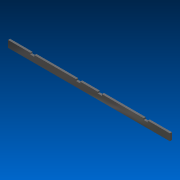
# Autodesk Inventor part: spacer 2
Saved by Autodesk Inventor 2012 (Build 160160000, 160)
## iProperties
Created: 2012-07-02
Part Number: spacer 2
Material: Default
Document SubType Name: Modeling
Designer: Hemant
Density: 1 g/cm^3
Author: Hemant
Autodesk Inventor part; units mm, degrees
ref_plane "YZ Plane" through (0, 0, 0) normal (1, 0, 0) x (0, 1, 0)
ref_plane "XZ Plane" through (0, 0, 0) normal (0, 1, 0) x (-1, 0, 0)
ref_plane "XY Plane" through (0, 0, 0) normal (0, 0, 1) x (1, 0, 0)
sketch "Sketch1" plane through (0, 0, 0) normal (0, 0, 1) x (1, 0, 0)
  line L0 (0, 0) -> (1003.3, 0)
  line L1 (1003.3, 0) -> (1003.3, 42.3672)
  line L2 (1003.3, 42.3672) -> (0, 42.3672)
  line L3 (0, 42.3672) -> (0, 0)
  dimension "d0" = 42.3672
  dimension "d1" = 1003.3
  constraints: 8 end point, 2 parallel, 1 horizontal, 1 perpendicular
  measures "d0" distance between parallel lines of L2 L0
  measures "d1" distance between parallel lines of L1 L3
extrude "Extrusion1" add sketch "Sketch1" against normal blind 12.7
sketch "Sketch2" plane through (0, 0, 0) normal (0, 0, 1) x (1, 0, 0)
  line L0 (1003.3, 0) -> (1003.3, 42.3672) projected
  line L1 (1003.3, 42.3672) -> (0, 42.3672) projected
  line L2 (0, 42.3672) -> (0, 0) projected
  line L3 (137.16, 42.3672) -> (162.56, 42.3672)
  line L4 (162.56, 42.3672) -> (162.56, 32.8422)
  line L5 (162.56, 32.8422) -> (137.16, 32.8422)
  line L6 (137.16, 32.8422) -> (137.16, 42.3672)
  line L7 (866.14, 42.3672) -> (840.74, 42.3672)
  line L8 (840.74, 42.3672) -> (840.74, 32.8422)
  line L9 (840.74, 32.8422) -> (866.14, 32.8422)
  line L10 (866.14, 32.8422) -> (866.14, 42.3672)
  line L11 (421.64, 42.3672) -> (447.04, 42.3672)
  line L12 (447.04, 42.3672) -> (447.04, 32.8422)
  line L13 (447.04, 32.8422) -> (421.64, 32.8422)
  line L14 (421.64, 32.8422) -> (421.64, 42.3672)
  line L15 (581.66, 42.3672) -> (556.26, 42.3672)
  line L16 (556.26, 42.3672) -> (556.26, 32.8422)
  line L17 (556.26, 32.8422) -> (581.66, 32.8422)
  line L18 (581.66, 32.8422) -> (581.66, 42.3672)
  dimension "d4" = 9.525
  dimension "d5" = 25.4
  dimension "d6" = 137.16
  dimension "d7" = 137.16
  dimension "d8" = 25.4
  dimension "d9" = 9.525
  dimension "d12" = 421.64
  dimension "d13" = 25.4
  dimension "d14" = 9.525
  dimension "d15" = 421.64
  dimension "d16" = 25.4
  dimension "d17" = 9.525
  constraints: 32 end point, 8 parallel, 4 horizontal, 4 perpendicular, 4 point on line
  measures "d4" distance between parallel lines of L1 L5
  measures "d5" distance between parallel lines of L4 L6
  measures "d6" distance between parallel lines of L6 L2
  measures "d7" distance between parallel lines of L10 L0
  measures "d8" distance between parallel lines of L8 L10
  measures "d9" distance between parallel lines of L1 L9
  measures "d12" distance from line of L11.start L2
  measures "d13" distance between parallel lines of L12 L14
  measures "d14" distance between parallel lines of L13 L1
  measures "d15" distance from line of L0 L15.start
  measures "d16" distance from line of L16 L15.start
  measures "d17" distance between parallel lines of L17 L1
extrude "Extrusion3" cut sketch "Sketch2" against normal blind 12.7
body "Solid1"
